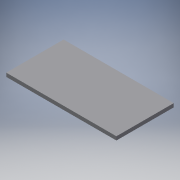
# Autodesk Inventor part: Back Plate
Saved by Autodesk Inventor 2016 (Build 200138000, 138)
## iProperties
Created: 2016-11-04
Part Number: Back Plate
Material: Generic
Document SubType Name: Modeling
Designer: william
Density: 1 g/cm^3
Appearance: Default
Author: william
Autodesk Inventor part; units mm, degrees
ref_plane "YZ Plane" through (0, 0, 0) normal (1, 0, 0) x (0, 1, 0)
ref_plane "XZ Plane" through (0, 0, 0) normal (0, 1, 0) x (-1, 0, 0)
ref_plane "XY Plane" through (0, 0, 0) normal (0, 0, 1) x (1, 0, 0)
sketch "Sketch1" plane through (0, 0, 0) normal (0, 0, 1) x (1, 0, 0)
  line L0 (0, 0) -> (192, 0)
  line L1 (192, 0) -> (192, 60)
  line L2 (192, 60) -> (0, 60)
  line L3 (0, 60) -> (0, 0)
  line L4 (192, 45) -> (186.8, 45)
  line L5 (186.8, 45) -> (186.8, 15)
  line L6 (186.8, 15) -> (192, 15)
  line L7 (192, 15) -> (192, 45)
  line L8 (0, 45) -> (5.2, 45)
  line L9 (5.2, 45) -> (5.2, 15)
  line L10 (5.2, 15) -> (0, 15)
  line L11 (0, 15) -> (0, 45)
  line L12 (142, 0) -> (50, 0)
  line L13 (50, 0) -> (50, 5.2)
  line L14 (50, 5.2) -> (142, 5.2)
  line L15 (142, 5.2) -> (142, 0)
  dimension "d0" = 60
  dimension "d1" = 192
  dimension "d4" = 5.2
  dimension "d5" = 30
  dimension "d6" = 15
  dimension "d7" = 30
  dimension "d8" = 5.2
  dimension "d9" = 15
  dimension "d12" = 50
  dimension "d13" = 50
  dimension "d14" = 5.2
  constraints: 32 end point, 8 parallel, 4 horizontal, 4 perpendicular, 3 point on line
  measures "d0" distance of L0.end L1.end
  measures "d1" distance of L1.end L2.end
  measures "d4" distance of L4.start L4.end
  measures "d5" distance of L4.end L5.end
  measures "d6" distance between parallel lines of L0 L6
  measures "d7" distance of L8.end L9.end
  measures "d8" distance of L8.start L8.end
  measures "d9" distance between parallel lines of L0 L10
  measures "d12" distance between parallel lines of L1 L15
  measures "d13" distance between parallel lines of L13 L3
  measures "d14" distance between parallel lines of L12 L14
extrude "Extrusion3" add sketch "Sketch1" along normal blind 5.2 contours L3 L10 L9 L8 L2 L1 L4 L5 L6 L0 L15 L14 L13
body "Solid3"
